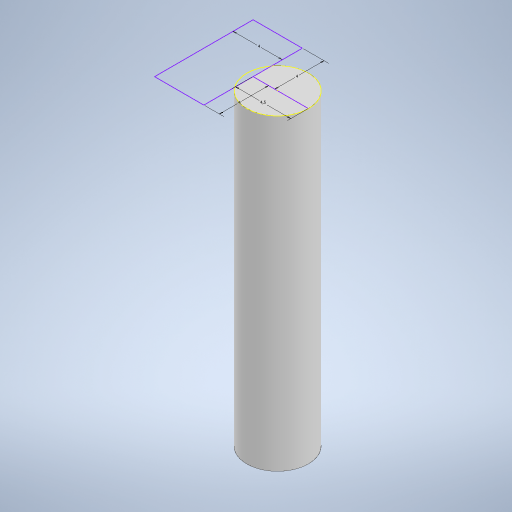
# Autodesk Inventor part: AXE
Saved by Autodesk Inventor 2024 (Build 280153000, 153)
## iProperties
Created: 2025-04-30
Part Number: AXE
Material: Generic
Document SubType Name: Modeling
Designer: Bjarni Heselmans
Density: 1 g/cm^3
Appearance: Default
Author: Bjarni Heselmans
Autodesk Inventor part; units mm, degrees
ref_plane "YZ Plane" through (0, 0, 0) normal (1, 0, 0) x (0, 1, 0)
ref_plane "XZ Plane" through (0, 0, 0) normal (0, 1, 0) x (-1, 0, 0)
ref_plane "XY Plane" through (0, 0, 0) normal (0, 0, 1) x (1, 0, 0)
sketch "Sketch1" plane through (0, 0, 0) normal (0, 0, 1) x (1, 0, 0)
  circle A0 centre (0, 0) radius 2.5
  dimension "d0" = 5
  constraints: 1 centre point, 1 coincident
  measures "d0" diameter of A0
extrude "Extrusion1" add sketch "Sketch1" along normal blind 25
sketch "Sketch2" plane through (0, 0, 25) normal (0, 0, 1) x (1, 0, 0)
  circle A0 centre (0, 0) radius 2.5 projected
  line L0 (2.5, 0) -> (-2, 0)
  line L1 (-2, 0) -> (-2, 4)
  line L2 (-2, 0) -> (-2, -4)
  line L3 (-2, -4) -> (-6, -4)
  line L4 (-6, -4) -> (-6, 4)
  line L5 (-6, 4) -> (-2, 4)
  point P0 (-2, -1.5)
  point P1 (-2, 1.5)
  dimension "d3" = 4.5
  dimension "d6" = 4
  dimension "d7" = 4
  dimension "d8" = 4
  constraints: 12 end point, 4 perpendicular, 1 horizontal, 1 vertical, 2 other
  measures "d3" distance of L0.start L0.end
  measures "d6" distance between parallel lines of L1 L4
  measures "d7" distance between parallel lines of L0 L5
  measures "d8" distance between parallel lines of L0 L3
extrude "Extrusion2" cut sketch "Sketch2" against normal blind 15 contours A0 L2 L3 L4 L5 L1
extrude "Extrusion3" cut sketch "Sketch2" against normal blind 15 contours L1 L2 A0
body "Solid1"
